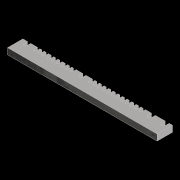
# Autodesk Inventor part: 3d_LM-Welding_Tooling - Top Comb
Saved by Autodesk Inventor 2018.3 (Build 223284000, 284)
## iProperties
Created: 2026-01-21
Part Number: 3d_LM-Welding_Tooling - Top Comb
Material: Steel, Carbon
Document SubType Name: Modeling
Designer: aca6
Density: 7.85 g/cm^3
Appearance: Semi-Polished
Author: aca6
Autodesk Inventor part; units mm, degrees
ref_plane "YZ Plane" through (0, 0, 0) normal (1, 0, 0) x (0, 1, 0)
ref_plane "XZ Plane" through (0, 0, 0) normal (0, 1, 0) x (-1, 0, 0)
sketch "Sketch1" plane through (0, 0, 0) normal (0, 0, 1) x (1, 0, 0)
  line L0 (-25.25, 2.5) -> (25.25, 2.5)
  line L1 (25.25, 2.5) -> (25.25, -2.5)
  line L2 (25.25, -2.5) -> (-25.25, -2.5)
  line L3 (-25.25, -2.5) -> (-25.25, 2.5)
  circle A0 centre (-22.5, 1.3) radius 0.5
  circle A1 centre (-19.4, 1.3) radius 0.4
  circle A2 centre (-10.4, 1.3) radius 0.4
  circle A3 centre (-18, 1.3) radius 0.4
  circle A4 centre (-13.5, 1.3) radius 0.4
  circle A5 centre (-16.6, 1.3) radius 0.4
  circle A6 centre (-14.9, 1.3) radius 0.4
  circle A7 centre (-12.1, 1.3) radius 0.4
  circle A8 centre (-7.6, 1.3) radius 0.4
  circle A9 centre (-9, 1.3) radius 0.4
  line L4 (0, 0) -> (0, 2.997) construction
  line L5 (0, 0) -> (1.9732, 0) construction
  circle A10 centre (-4.5, 1.3) radius 0.5
  circle A11 centre (-1.5, 1.3) radius 0.4
  circle A12 centre (0, 1.3) radius 0.4
  circle A13 centre (1.5, 1.3) radius 0.4
  circle A14 centre (3, 1.3) radius 0.4
  circle A15 centre (4.5, 1.3) radius 0.4
  circle A16 centre (6, 1.3) radius 0.4
  circle A17 centre (7.5, 1.3) radius 0.4
  circle A18 centre (9, 1.3) radius 0.4
  circle A19 centre (10.5, 1.3) radius 0.4
  circle A20 centre (12, 1.3) radius 0.4
  circle A21 centre (13.5, 1.3) radius 0.4
  circle A22 centre (15, 1.3) radius 0.4
  circle A23 centre (18, 1.3) radius 0.625
  circle A24 centre (22.5, 1.3) radius 0.625
  line L6 (-22, 1.3) -> (-22, 2.5)
  line L7 (-23, 1.3) -> (-23, 2.5)
  line L8 (-19, 1.3) -> (-19, 2.5)
  line L9 (-19.8, 1.3) -> (-19.8, 2.5)
  line L10 (-17.6, 1.3) -> (-17.6, 2.5)
  line L11 (-18.4, 1.3) -> (-18.4, 2.5)
  line L12 (-16.2, 1.3) -> (-16.2, 2.5)
  line L13 (-17, 1.3) -> (-17, 2.5)
  line L14 (-14.5, 1.3) -> (-14.5, 2.5)
  line L15 (-15.3, 1.3) -> (-15.3, 2.5)
  line L16 (-13.1, 1.3) -> (-13.1, 2.5)
  line L17 (-13.9, 1.3) -> (-13.9, 2.5)
  line L18 (-11.7, 1.3) -> (-11.7, 2.5)
  line L19 (-12.5, 1.3) -> (-12.5, 2.5)
  line L20 (-10, 1.3) -> (-10, 2.5)
  line L21 (-10.8, 1.3) -> (-10.8, 2.5)
  line L22 (-8.6, 1.3) -> (-8.6, 2.5)
  line L23 (-9.4, 1.3) -> (-9.4, 2.5)
  line L24 (-7.2, 1.3) -> (-7.2, 2.5)
  line L25 (-8, 1.3) -> (-8, 2.5)
  line L26 (-4, 1.3) -> (-4, 2.5)
  line L27 (-5, 1.3) -> (-5, 2.5)
  line L28 (-1.1, 1.3) -> (-1.1, 2.5)
  line L29 (-1.9, 1.3) -> (-1.9, 2.5)
  line L30 (0.4, 1.3) -> (0.4, 2.5)
  line L31 (-0.4, 1.3) -> (-0.4, 2.5)
  line L32 (1.9, 1.3) -> (1.9, 2.5)
  line L33 (1.1, 1.3) -> (1.1, 2.5)
  line L34 (2.6, 1.3) -> (2.6, 2.5)
  line L35 (3.4, 1.3) -> (3.4, 2.5)
  line L36 (4.1, 1.3) -> (4.1, 2.5)
  line L37 (4.9, 1.3) -> (4.9, 2.5)
  line L38 (5.6, 1.3) -> (5.6, 2.5)
  line L39 (6.4, 1.3) -> (6.4, 2.5)
  line L40 (7.1, 1.3) -> (7.1, 2.5)
  line L41 (7.9, 1.3) -> (7.9, 2.5)
  line L42 (8.6, 1.3) -> (8.6, 2.5)
  line L43 (9.4, 1.3) -> (9.4, 2.5)
  line L44 (10.1, 1.3) -> (10.1, 2.5)
  line L45 (10.9, 1.3) -> (10.9, 2.5)
  line L46 (11.6, 1.3) -> (11.6, 2.5)
  line L47 (12.4, 1.3) -> (12.4, 2.5)
  line L48 (13.1, 1.3) -> (13.1, 2.5)
  line L49 (13.9, 1.3) -> (13.9, 2.5)
  line L50 (14.6, 1.3) -> (14.6, 2.5)
  line L51 (15.4, 1.3) -> (15.4, 2.5)
  line L52 (17.375, 1.3) -> (17.375, 2.5)
  line L53 (18.625, 1.3) -> (18.625, 2.5)
  line L54 (23.125, 1.3) -> (23.125, 2.5)
  line L55 (21.875, 1.3) -> (21.875, 2.5)
  circle A25 centre (22.5, -1.3) radius 0.625
  circle A26 centre (18, -1.3) radius 0.625
  circle A27 centre (15, -1.3) radius 0.4
  circle A28 centre (13.5, -1.3) radius 0.4
  circle A29 centre (12, -1.3) radius 0.4
  circle A30 centre (10.5, -1.3) radius 0.4
  circle A31 centre (9, -1.3) radius 0.4
  circle A32 centre (7.5, -1.3) radius 0.4
  circle A33 centre (6, -1.3) radius 0.4
  circle A34 centre (4.5, -1.3) radius 0.4
  circle A35 centre (3, -1.3) radius 0.4
  circle A36 centre (1.5, -1.3) radius 0.4
  circle A37 centre (0, -1.3) radius 0.4
  circle A38 centre (-1.5, -1.3) radius 0.4
  circle A39 centre (-7.5, -1.3) radius 0.4
  circle A40 centre (-9, -1.3) radius 0.4
  circle A41 centre (-10.5, -1.3) radius 0.4
  circle A42 centre (-12.6, -1.3) radius 0.4
  circle A43 centre (-14.4, -1.3) radius 0.4
  circle A44 centre (-16.5, -1.3) radius 0.4
  circle A45 centre (-18, -1.3) radius 0.4
  circle A46 centre (-19.5, -1.3) radius 0.4
  circle A47 centre (-21.6, -1.3) radius 0.4
  circle A48 centre (-23.4, -1.3) radius 0.4
  line L56 (23.125, -1.3) -> (23.125, -2.5)
  line L57 (21.875, -1.3) -> (21.875, -2.5)
  line L58 (18.625, -1.3) -> (18.625, -2.5)
  line L59 (17.375, -1.3) -> (17.375, -2.5)
  line L60 (15.4, -1.3) -> (15.4, -2.5)
  line L61 (14.6, -1.3) -> (14.6, -2.5)
  line L62 (13.9, -1.3) -> (13.9, -2.5)
  line L63 (13.1, -1.3) -> (13.1, -2.5)
  line L64 (12.4, -1.3) -> (12.4, -2.5)
  line L65 (11.6, -1.3) -> (11.6, -2.5)
  line L66 (10.9, -1.3) -> (10.9, -2.5)
  line L67 (10.1, -1.3) -> (10.1, -2.5)
  line L68 (9.4, -1.3) -> (9.4, -2.5)
  line L69 (8.6, -1.3) -> (8.6, -2.5)
  line L70 (7.9, -1.3) -> (7.9, -2.5)
  line L71 (7.1, -1.3) -> (7.1, -2.5)
  line L72 (6.4, -1.3) -> (6.4, -2.5)
  line L73 (5.6, -1.3) -> (5.6, -2.5)
  line L74 (4.9, -1.3) -> (4.9, -2.5)
  line L75 (4.1, -1.3) -> (4.1, -2.5)
  line L76 (3.4, -1.3) -> (3.4, -2.5)
  line L77 (2.6, -1.3) -> (2.6, -2.5)
  line L78 (1.9, -1.3) -> (1.9, -2.5)
  line L79 (1.1, -1.3) -> (1.1, -2.5)
  line L80 (0.4, -1.3) -> (0.4, -2.5)
  line L81 (-0.4, -1.3) -> (-0.4, -2.5)
  line L82 (-1.9, -1.3) -> (-1.9, -2.5)
  line L83 (-1.1, -1.3) -> (-1.1, -2.5)
  line L84 (-7.9, -1.3) -> (-7.9, -2.5)
  line L85 (-7.1, -1.3) -> (-7.1, -2.5)
  line L86 (-8.6, -1.3) -> (-8.6, -2.5)
  line L87 (-9.4, -1.3) -> (-9.4, -2.5)
  line L88 (-10.1, -1.3) -> (-10.1, -2.5)
  line L89 (-10.9, -1.3) -> (-10.9, -2.5)
  line L90 (-12.2, -1.3) -> (-12.2, -2.5)
  line L91 (-13, -1.3) -> (-13, -2.5)
  line L92 (-14, -1.3) -> (-14, -2.5)
  line L93 (-14.8, -1.3) -> (-14.8, -2.5)
  line L94 (-16.1, -1.3) -> (-16.1, -2.5)
  line L95 (-16.9, -1.3) -> (-16.9, -2.5)
  line L96 (-17.6, -1.3) -> (-17.6, -2.5)
  line L97 (-18.4, -1.3) -> (-18.4, -2.5)
  line L98 (-19.1, -1.3) -> (-19.1, -2.5)
  line L99 (-19.9, -1.3) -> (-19.9, -2.5)
  line L100 (-21.2, -1.3) -> (-21.2, -2.5)
  line L101 (-22, -1.3) -> (-22, -2.5)
  line L102 (-23, -1.3) -> (-23, -2.5)
  line L103 (-23.8, -1.3) -> (-23.8, -2.5)
  dimension "d0" = 50.5
  dimension "d1" = 5
  dimension "d3" = 1
  dimension "d4" = 2.75
  dimension "d5" = 0.8
  dimension "d6" = 0.8
  dimension "d7" = 0.8
  dimension "d8" = 0.8
  dimension "d9" = 0.8
  dimension "d10" = 0.8
  dimension "d11" = 0.8
  dimension "d12" = 0.8
  dimension "d13" = 0.8
  dimension "d14" = 3.1
  dimension "d15" = 1.4
  dimension "d16" = 1.4
  dimension "d17" = 1.4
  dimension "d18" = 1.4
  dimension "d19" = 1.7
  dimension "d20" = 1.4
  dimension "d21" = 1.4
  dimension "d22" = 1.7
  dimension "d23" = 1.2
  dimension "d24" = 1
  dimension "d25" = 3.1
  dimension "d26" = 0.8
  dimension "d27" = 0.8
  dimension "d28" = 0.8
  dimension "d29" = 0.8
  dimension "d30" = 0.8
  dimension "d31" = 0.8
  dimension "d32" = 0.8
  dimension "d33" = 0.8
  dimension "d34" = 0.8
  dimension "d35" = 0.8
  dimension "d36" = 0.8
  dimension "d37" = 0.8
  dimension "d38" = 3
  dimension "d39" = 1.5
  dimension "d40" = 1.5
  dimension "d41" = 1.5
  dimension "d42" = 1.5
  dimension "d43" = 1.5
  dimension "d44" = 1.5
  dimension "d45" = 1.5
  dimension "d46" = 1.5
  dimension "d47" = 1.5
  dimension "d48" = 1.5
  dimension "d49" = 1.5
  dimension "d50" = 1.25
  dimension "d51" = 1.25
  dimension "d52" = 3
  dimension "d53" = 4.5
  dimension "d121" = 1.25
  dimension "d122" = 1.25
  dimension "d125" = 0.8
  dimension "d126" = 0.8
  dimension "d127" = 0.8
  dimension "d128" = 0.8
  dimension "d129" = 0.8
  dimension "d130" = 0.8
  dimension "d131" = 0.8
  dimension "d132" = 0.8
  dimension "d133" = 0.8
  constraints: 204 end point, 98 point on circle, 98 tangent, 92 vertical, 49 centre point, 47 horizontal alignment, 10 parallel, 3 horizontal, 107 other
  measures "d0" distance of L3.end L1.start
  measures "d1" distance of L3.start L3.end
  measures "d3" diameter of A0
  measures "d4" distance from line of L3 A0.centre
  measures "d5" diameter of A1
  measures "d6" diameter of A2
  measures "d7" diameter of A3
  measures "d8" diameter of A4
  measures "d9" diameter of A5
  measures "d10" diameter of A6
  measures "d11" diameter of A7
  measures "d12" diameter of A8
  measures "d13" diameter of A9
  measures "d14" distance of A1.centre A0.centre
  measures "d15" distance of A3.centre A1.centre
  measures "d16" distance of A5.centre A3.centre
  measures "d17" distance of A4.centre A6.centre
  measures "d18" distance of A4.centre A7.centre
  measures "d19" distance of A6.centre A5.centre
  measures "d20" distance of A9.centre A2.centre
  measures "d21" distance of A8.centre A9.centre
  measures "d22" distance of A2.centre A7.centre
  measures "d24" diameter of A10
  measures "d25" distance of A10.centre A8.centre
  measures "d26" diameter of A11
  measures "d27" diameter of A12
  measures "d28" diameter of A13
  measures "d29" diameter of A14
  measures "d30" diameter of A15
  measures "d31" diameter of A16
  measures "d32" diameter of A17
  measures "d33" diameter of A18
  measures "d34" diameter of A19
  measures "d35" diameter of A20
  measures "d36" diameter of A21
  measures "d37" diameter of A22
  measures "d38" distance of A11.centre A10.centre
  measures "d39" distance of A12.centre A11.centre
  measures "d40" distance of A13.centre A12.centre
  measures "d41" distance of A14.centre A13.centre
  measures "d42" distance of A14.centre A15.centre
  measures "d43" distance of A16.centre A15.centre
  measures "d44" distance of A17.centre A16.centre
  measures "d45" distance of A18.centre A17.centre
  measures "d46" distance of A18.centre A19.centre
  measures "d47" distance of A20.centre A19.centre
  measures "d48" distance of A21.centre A20.centre
  measures "d49" distance of A22.centre A21.centre
  measures "d50" diameter of A23
  measures "d51" diameter of A24
  measures "d52" distance of A23.centre A22.centre
  measures "d53" distance of A24.centre A23.centre
  measures "d121" diameter of A25
  measures "d122" diameter of A26
  measures "d125" diameter of A27
  measures "d126" diameter of A28
  measures "d127" diameter of A29
  measures "d128" diameter of A30
  measures "d129" diameter of A31
  measures "d130" diameter of A32
  measures "d131" diameter of A33
  measures "d132" diameter of A34
  measures "d133" diameter of A35
extrude "Extrusion1" add sketch "Sketch1" along normal blind 2 contours L0 L7 A0 L6 L9 A1 L8 L11 A3 L10 L13 A5 L12 L15 A6 L14 L17 A4 L16 L19 A7 L18 L21 A2 L20 L23 A9 L22 L25 A8 L24 L27 A10 L26 L29 A11 L28 L31 A12 L30 L33 A13 L32 L34 A14 L35 L36 A15 L37 L38 A16 L39 L40 A17 L41 L42 A18 L43 L44 A19 L45 L46 A20 L47 L48 A21 L49 L50 A22 L51 L52 A23 L53 L55 A24 L54 L1 L2 L56 A25 L57 L58 A26 L59 L60 A27 L61 L62 A28 L63 L64 A29 L65 L66 A30 L67 L68 A31 L69 L70 A32 L71 L72 A33 L73 L74 A34 L75 L76 A35 L77 L78 A36 L79 L80 A37 L81 L83 A38 L82 L85 A39 L84 L86 A40 L87 L88 A41 L89 L90 A42 L91 L92 A43 L93 L94 A44 L95 L96 A45 L97 L98 A46 L99 L100 A47 L101 L102 A48 L103 L3
ref_plane "Work Plane1" through (-26.5, -2, 0) normal (-1, 0, 0) x (0, 0, 1)
sketch "Sketch12" plane through (0, 0, 0) normal (0, 0, -1) x (-1, 0, 0)
  arc A0 (-24.0126, -0.5173) -> (-23.9919, 1.0846) centre (-25.2704, 0.3) ccw projected
  arc A1 (-24.2504, 2) -> (-23.9919, 1.0846) centre (-22.5004, 2) ccw projected
  arc A2 (-24.0126, -0.5173) -> (-24.2331, -2) centre (-22.5004, -1.5) ccw projected
  line L0 (-24.2331, -2) -> (-25.0004, -2) projected
  line L1 (-25.0004, 2) -> (-24.2504, 2) projected
  line L2 (-25.0004, -2.1) -> (-24.0947, -2.1)
  arc A3 (-23.9286, -0.5716) -> (-23.8794, -2.5) centre (-22.5004, -1.5) ccw
  arc A4 (-23.9286, -0.5716) -> (-23.9067, 1.1369) centre (-25.2704, 0.3) ccw
  arc A5 (-24.1474, 2.1) -> (-23.9067, 1.1369) centre (-22.5004, 2) ccw
  line L3 (-24.1474, 2.1) -> (-25, 2.1)
  line L4 (-24.1474, 2.1) -> (-24.1474, 2.5)
  line L5 (-25.25, 2.5) -> (-23.125, 2.5) projected
  line L6 (-24.1474, 2.5) -> (-25.25, 2.5)
  line L7 (-23.125, -2.5) -> (-25.25, -2.5) projected
  line L8 (-25.25, 2.5) -> (-25.25, -2.5)
  line L9 (-25.25, -2.5) -> (-24.0947, -2.5)
  line L10 (-24.0947, -2.1) -> (-24.0947, -2.5)
  point P0 (0, 0)
  dimension "d188" = 0.1
  constraints: 14 end point, 7 point on circle, 3 centre point, 2 perpendicular, 2 point on line, 1 collinear, 1 vertical, 2 other
  measures "d188" radial gap between concentric circles of A1 A5
extrude "Extrusion12" cut sketch "Sketch12" against normal blind 10
sketch "Sketch13" plane through (0, 0, 0) normal (0, 0, -1) x (-1, 0, 0)
  arc A0 (24.3834, 0.9639) -> (24.3834, -0.9639) centre (26.1358, 0) ccw projected
  arc A1 (24.3834, 0.9639) -> (24.6496, 2) centre (22.4996, 2) ccw projected
  arc A2 (24.6496, -2) -> (24.3834, -0.9639) centre (22.4996, -2) ccw projected
  line L0 (24.6496, -2) -> (25, -2) projected
  line L1 (24.9996, 2) -> (24.6496, 2) projected
  line L2 (24.6496, 2) -> (24.6496, 2.5)
  line L3 (23, 2.5) -> (25.25, 2.5) projected
  line L4 (24.6496, -2) -> (24.6496, -2.5)
  line L5 (25.25, -2.5) -> (23.8, -2.5) projected
  line L6 (24.6496, -2.5) -> (25.25, -2.5)
  line L7 (25.25, -2.5) -> (25.25, 2.5)
  line L8 (25.25, 2.5) -> (25.25, -2.5) projected
  line L9 (25.25, 2.5) -> (24.6496, 2.5)
  line L10 (25, -2.1) -> (24.5471, -2.1)
  arc A3 (24.5471, -2.1) -> (24.2958, -1.012) centre (22.4996, -2) ccw
  arc A4 (24.2958, 1.012) -> (24.2958, -1.012) centre (26.1358, 0) ccw
  arc A5 (24.2958, 1.012) -> (24.5471, 2.1) centre (22.4996, 2) ccw
  line L11 (24.5471, 2.1) -> (25, 2.1)
  line L12 (24.55, -2.6) -> (25.35, -2.6)
  line L13 (25.35, -2.6) -> (25.35, 2.6)
  line L14 (25.35, 2.6) -> (24.55, 2.6)
  line L15 (24.5471, -2.5) -> (24.6496, -2.5)
  line L16 (24.6496, 2.5) -> (24.5471, 2.5)
  line L17 (24.5471, 2.1) -> (24.5471, 2.5)
  line L18 (24.5471, 2.5) -> (24.6496, 2.5)
  line L19 (24.5471, -2.1) -> (24.5471, -2.5)
  line L20 (24.5471, -2.5) -> (24.6496, -2.5)
  point P0 (0, 0)
  dimension "d193" = 0.1
  constraints: 32 end point, 6 point on circle, 5 point on line, 4 collinear, 3 centre point, 3 perpendicular, 3 vertical, 6 other
  measures "d193" radial gap between concentric circles of A0 A4
extrude "Extrusion13" cut sketch "Sketch13" against normal blind 10
sketch "Sketch14" plane through (0, 0, 0) normal (0, 0, -1) x (-1, 0, 0)
  arc A0 (6.3296, -2) -> (4.9596, -2) centre (5.6446, -2) ccw projected
  arc A1 (4.9596, -2) -> (6.3296, -2) centre (5.6446, -2) ccw projected
  arc A2 (4.0396, -2) -> (2.6696, -2) centre (3.3546, -2) ccw projected
  arc A3 (2.6696, -2) -> (4.0396, -2) centre (3.3546, -2) ccw projected
  arc A4 (4.1396, -2) -> (2.5696, -2) centre (3.3546, -2) ccw
  arc A5 (2.5696, -2) -> (4.1396, -2) centre (3.3546, -2) ccw
  arc A6 (6.4296, -2) -> (4.8596, -2) centre (5.6446, -2) ccw
  arc A7 (4.8596, -2) -> (6.4296, -2) centre (5.6446, -2) ccw
  point P0 (0, 0)
  dimension "d195" = 0.1
  dimension "d196" = 0.1
  constraints: 8 point on circle, 4 centre point, 2 other
  measures "d195" radial gap between concentric circles of A2 A4
  measures "d196" radial gap between concentric circles of A0 A6
extrude "Extrusion14" cut sketch "Sketch14" against normal blind 10 contours A1 A0 | A3 A2 | A5 A4 | A7 A6
sketch "Sketch15" plane through (0, 0, 2) normal (0, 0, 1) x (1, 0, 0)
  line L0 (-23.8, -0.675) -> (23.125, -0.675)
  line L1 (23.125, -0.675) -> (23.125, -2.5)
  line L2 (23.125, -2.5) -> (-23.8, -2.5)
  line L3 (-23.8, -2.5) -> (-23.8, -0.675)
  line L4 (-23.8, -2.5) -> (-23.8, -1.3) projected
  line L5 (23.125, -1.3) -> (23.125, -2.5) projected
  line L6 (18.625, -2.5) -> (21.875, -2.5) projected
  arc A0 (23.125, -1.3) -> (21.875, -1.3) centre (22.5, -1.3) ccw projected
  line L7 (-24.5471, -2.5) -> (-23.8, -2.5) projected
  line L8 (-24.5496, 2.5) -> (-23.8, 2.5)
  line L9 (-23.8, 2.5) -> (-23.8, -2.5)
  line L10 (-23.8, -2.5) -> (-24.5496, -2.5)
  line L11 (24.2038, 2.5) -> (23.125, 2.5)
  line L12 (23.125, 2.5) -> (23.125, -2.5)
  line L13 (23.125, -2.5) -> (24.2038, -2.5)
  arc A1 (23.8794, -2.5) -> (23.9286, -0.5716) centre (22.5004, -1.5) ccw projected
  line L14 (-24.5496, 2.5117) -> (-24.5496, -2.5071)
  arc A2 (-24.2958, -1.012) -> (-24.5471, -2.1) centre (-22.4996, -2) ccw projected
  line L15 (24.2038, -2.5071) -> (24.2038, 2.5117)
  point P0 (0, 0)
  point P1 (-23.8, -1.9)
  point P2 (23.125, -1.9)
  point P3 (20.25, -2.5)
  point P4 (22.5, -0.675)
  point P5 (24.1474, 2.5)
  constraints: 24 end point, 9 point on line, 4 parallel, 3 horizontal, 3 midpoint, 3 perpendicular, 2 tangent, 2 vertical, 1 point on circle
extrude "Extrusion15" add sketch "Sketch15" against normal up to surface (2 mm away)
body "Solid1"
